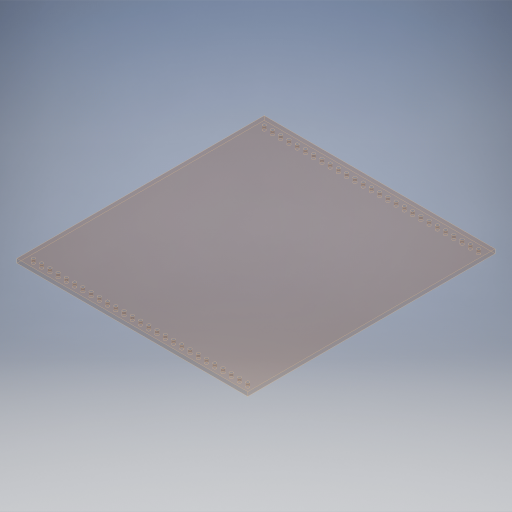
# Autodesk Inventor part: Polycarbonate-Note-Rest
Saved by Autodesk Inventor 2024.2 (Build 282272000, 272)
## iProperties
Created: 2024-01-23
Part Number: Polycarbonate-Note-Rest
Material: Polycarbonate, Smoke
Document SubType Name: Modeling
Designer: rohan
Density: 1.2 g/cm^3
Appearance: Polycarbonate - Smoked
Author: rohan
Autodesk Inventor part; units mm, degrees
ref_plane "YZ Plane" through (0, 0, 0) normal (1, 0, 0) x (0, 1, 0)
ref_plane "XZ Plane" through (0, 0, 0) normal (0, 1, 0) x (-1, 0, 0)
ref_plane "XY Plane" through (0, 0, 0) normal (0, 0, 1) x (1, 0, 0)
sketch "Sketch4" plane through (0, 0, 0) normal (0, 1, 0) x (-1, 0, 0)
  line L0 (-177.8, 190.5) -> (177.8, 190.5)
  line L1 (177.8, 190.5) -> (177.8, -190.5)
  line L2 (177.8, -190.5) -> (-177.8, -190.5)
  line L3 (-177.8, -190.5) -> (-177.8, 190.5)
  line L4 (-177.8, 190.5) -> (177.8, -190.5) construction
  line L5 (177.8, 190.5) -> (-177.8, -190.5) construction
  circle A0 centre (165.1, 177.8) radius 2.4892
  circle A1 centre (152.4, 177.8) radius 2.4892
  circle A2 centre (139.7, 177.8) radius 2.4892
  circle A3 centre (127, 177.8) radius 2.4892
  circle A4 centre (114.3, 177.8) radius 2.4892
  circle A5 centre (101.6, 177.8) radius 2.4892
  circle A6 centre (88.9, 177.8) radius 2.4892
  circle A7 centre (76.2, 177.8) radius 2.4892
  circle A8 centre (63.5, 177.8) radius 2.4892
  circle A9 centre (50.8, 177.8) radius 2.4892
  circle A10 centre (38.1, 177.8) radius 2.4892
  circle A11 centre (25.4, 177.8) radius 2.4892
  circle A12 centre (12.7, 177.8) radius 2.4892
  circle A13 centre (0, 177.8) radius 2.4892
  circle A14 centre (-12.7, 177.8) radius 2.4892
  circle A15 centre (-25.4, 177.8) radius 2.4892
  circle A16 centre (-38.1, 177.8) radius 2.4892
  circle A17 centre (-50.8, 177.8) radius 2.4892
  circle A18 centre (-63.5, 177.8) radius 2.4892
  circle A19 centre (-76.2, 177.8) radius 2.4892
  circle A20 centre (-88.9, 177.8) radius 2.4892
  circle A21 centre (-101.6, 177.8) radius 2.4892
  circle A22 centre (-114.3, 177.8) radius 2.4892
  circle A23 centre (-127, 177.8) radius 2.4892
  circle A24 centre (-139.7, 177.8) radius 2.4892
  circle A25 centre (-152.4, 177.8) radius 2.4892
  circle A26 centre (-165.1, 177.8) radius 2.4892
  circle A27 centre (165.1, -177.8) radius 2.4892
  circle A28 centre (152.4, -177.8) radius 2.4892
  circle A29 centre (139.7, -177.8) radius 2.4892
  circle A30 centre (127, -177.8) radius 2.4892
  circle A31 centre (114.3, -177.8) radius 2.4892
  circle A32 centre (101.6, -177.8) radius 2.4892
  circle A33 centre (88.9, -177.8) radius 2.4892
  circle A34 centre (76.2, -177.8) radius 2.4892
  circle A35 centre (63.5, -177.8) radius 2.4892
  circle A36 centre (50.8, -177.8) radius 2.4892
  circle A37 centre (38.1, -177.8) radius 2.4892
  circle A38 centre (25.4, -177.8) radius 2.4892
  circle A39 centre (12.7, -177.8) radius 2.4892
  circle A40 centre (0, -177.8) radius 2.4892
  circle A41 centre (-12.7, -177.8) radius 2.4892
  circle A42 centre (-25.4, -177.8) radius 2.4892
  circle A43 centre (-38.1, -177.8) radius 2.4892
  circle A44 centre (-50.8, -177.8) radius 2.4892
  circle A45 centre (-63.5, -177.8) radius 2.4892
  circle A46 centre (-76.2, -177.8) radius 2.4892
  circle A47 centre (-88.9, -177.8) radius 2.4892
  circle A48 centre (-101.6, -177.8) radius 2.4892
  circle A49 centre (-114.3, -177.8) radius 2.4892
  circle A50 centre (-127, -177.8) radius 2.4892
  circle A51 centre (-139.7, -177.8) radius 2.4892
  circle A52 centre (-152.4, -177.8) radius 2.4892
  circle A53 centre (-165.1, -177.8) radius 2.4892
  point P0 (0, 0)
  dimension "d18" = 355.6
  dimension "d19" = 381
  dimension "d20" = 4.9784
  dimension "d21" = 12.7
  dimension "d22" = 12.7
  dimension "d25" = 12.7
  dimension "d28" = 355.6
  constraints: 54 centre point, 12 end point, 2 horizontal, 2 midpoint, 2 parallel, 1 perpendicular, 1 vertical, 106 other
  measures "d18" distance of L1.end L2.end
  measures "d19" distance of L0.end L1.end
  measures "d20" diameter of A0
  measures "d21" distance from line of L1 A0.centre
  measures "d22" distance from line of L0 A0.centre
  measures "d25" distance of A0.centre A1.centre
  measures "d28" distance of A0.centre A27.centre
extrude "Extrusion4" add sketch "Sketch4" along normal blind 6.35
body "Solid2"
